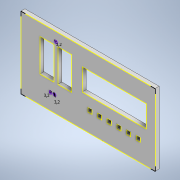
# Autodesk Inventor part: top
Saved by Autodesk Inventor 2021 (Build 250183000, 183)
## iProperties
Created: 2022-05-06
Part Number: top
Material: Všeobecné
Document SubType Name: Modeling
Designer: herman
Density: 1 g/cm^3
Appearance: Výchozí
Author: herman
Autodesk Inventor part; units mm, degrees
ref_plane "YZ Plane" through (0, 0, 0) normal (1, 0, 0) x (0, 1, 0)
ref_plane "XZ Plane" through (0, 0, 0) normal (0, 1, 0) x (-1, 0, 0)
ref_plane "XY Plane" through (0, 0, 0) normal (0, 0, 1) x (1, 0, 0)
sketch "Náčrt1" plane through (0, 0, 0) normal (0, 0, 1) x (1, 0, 0)
  line L0 (0, 75) -> (0, 5) projected
  line L1 (145, 80) -> (5, 80) projected
  line L2 (5, 0) -> (145, 0) projected
  line L3 (150, 5) -> (150, 75) projected
  line L4 (21.25, 29.75) -> (21.25, 66.25) projected
  line L5 (21.25, 66.25) -> (36.75, 66.25) projected
  line L6 (36.75, 66.25) -> (36.75, 29.75) projected
  line L7 (36.75, 29.75) -> (21.25, 29.75) projected
  line L8 (41.25, 29.75) -> (41.25, 66.25) projected
  line L9 (56.75, 29.75) -> (41.25, 29.75) projected
  line L10 (56.75, 66.25) -> (56.75, 29.75) projected
  line L11 (41.25, 66.25) -> (56.75, 66.25) projected
  line L12 (140, 36) -> (68.5, 36) projected
  line L13 (68.5, 36) -> (68.5, 60.5) projected
  line L14 (68.5, 60.5) -> (140, 60.5) projected
  line L15 (140, 60.5) -> (140, 36) projected
  line L16 (74.75, 19.75) -> (74.75, 24.25) projected
  line L17 (79.25, 24.25) -> (79.25, 19.75) projected
  line L18 (74.75, 24.25) -> (79.25, 24.25) projected
  line L19 (79.25, 19.75) -> (74.75, 19.75) projected
  line L20 (90.05, 19.75) -> (85.55, 19.75) projected
  line L21 (85.55, 19.75) -> (85.55, 24.25) projected
  line L22 (85.55, 24.25) -> (90.05, 24.25) projected
  line L23 (90.05, 24.25) -> (90.05, 19.75) projected
  line L24 (96.24, 19.75) -> (96.24, 24.25) projected
  line L25 (96.24, 24.25) -> (100.74, 24.25) projected
  line L26 (100.74, 19.75) -> (96.24, 19.75) projected
  line L27 (100.74, 24.25) -> (100.74, 19.75) projected
  line L28 (107.14, 19.75) -> (107.14, 24.25) projected
  line L29 (107.14, 24.25) -> (111.64, 24.25) projected
  line L30 (111.64, 19.75) -> (107.14, 19.75) projected
  line L31 (111.64, 24.25) -> (111.64, 19.75) projected
  line L32 (117.93, 19.75) -> (117.93, 24.25) projected
  line L33 (117.93, 24.25) -> (122.43, 24.25) projected
  line L34 (122.43, 19.75) -> (117.93, 19.75) projected
  line L35 (122.43, 24.25) -> (122.43, 19.75) projected
  line L36 (128.74, 19.75) -> (128.74, 24.25) projected
  line L37 (128.74, 24.25) -> (133.24, 24.25) projected
  line L38 (133.24, 19.75) -> (128.74, 19.75) projected
  line L39 (133.24, 24.25) -> (133.24, 19.75) projected
  circle A0 centre (38.995, 70.0066) radius 1.6
  circle A1 centre (33.0004, 18.0056) radius 1.6
  circle A2 centre (37.518, 18.0056) radius 1.6
  line L40 (5, 80) -> (0, 80)
  line L41 (0, 80) -> (0, 75)
  line L42 (0, 5) -> (0, 0)
  line L43 (0, 0) -> (5, 0)
  line L44 (145, 0) -> (150, 0)
  line L45 (150, 0) -> (150, 5)
  line L46 (150, 75) -> (150, 80)
  line L47 (145, 80) -> (150, 80)
  dimension "d0" = 3.2
  dimension "d1" = 3.2
  dimension "d2" = 3.2
  constraints: 16 end point, 4 perpendicular, 3 centre point, 3 point on line, 1 horizontal, 1 vertical
  measures "d0" diameter of A0
  measures "d1" diameter of A1
  measures "d2" diameter of A2
extrude "Vysunutí1" add sketch "Náčrt1" against normal blind 4.5
